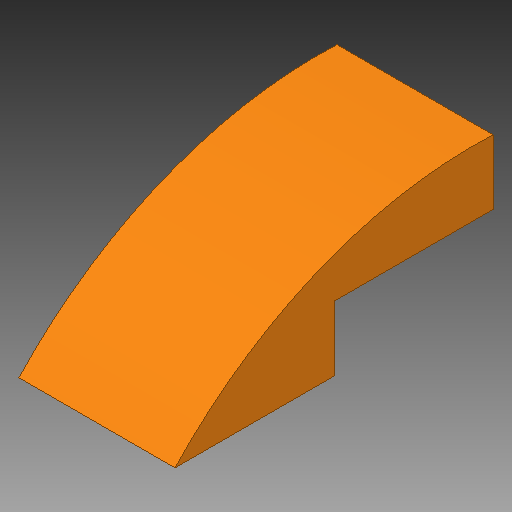
# Autodesk Inventor part: 2x1 curve
Saved by Autodesk Inventor 2017 (Build 210142000, 142)
## iProperties
Created: 2018-05-17
Part Number: 2x1 curve
Material: ABS Plastic
Document SubType Name: Modeling
Designer: 20000650
Density: 1.06 g/cm^3
Appearance: Orange
Mass: 0.311158 g
Surface Area: 4.69388 cm^2
Volume: 0.293546 cm^3
Author: 20000650
Autodesk Inventor part; units mm, degrees
ref_plane "YZ Plane" through (0, 0, 0) normal (1, 0, 0) x (0, 1, 0)
ref_plane "XZ Plane" through (0, 0, 0) normal (0, 1, 0) x (-1, 0, 0)
sketch "Sketch1" plane through (0, 0, 0) normal (1, 0, 0) x (0, 1, 0)
  line L0 (0, 0) -> (0, -7.9426)
  line L1 (0, -7.9426) -> (3.236, -7.9426)
  line L2 (3.236, -7.9426) -> (3.236, -15.8852)
  line L3 (3.236, -15.8852) -> (6.4618, -15.8852)
  arc A0 (6.4618, -15.8852) -> (0, 0) centre (-13.924, -14.9208) ccw
  dimension "d0" = 7.9426
  dimension "d1" = 3.236
  dimension "d2" = 7.9426
  dimension "d3" = 3.2258
  constraints: 8 end point, 3 perpendicular, 2 point on circle, 1 centre point, 1 vertical
  measures "d0" distance of L0.start L0.end
  measures "d1" distance of L0.end L1.end
  measures "d2" distance of L1.end L2.end
  measures "d3" distance of L2.end L3.end
extrude "Extrusion1" add sketch "Sketch1" along normal blind 7.7978
shell "Shell1" thickness 1.4732 removed faces 1 at (2.5993, 0, -2.6475)
ref_plane "Work Plane1" through (1.4732, 0, 0) normal (-1, 0, 0) x (0, 0, 1)
sketch "Sketch4" plane through (1.4732, 0, 0) normal (-1, 0, 0) x (0, 0, 1)
  line L0 (-7.9426, 3.236) -> (-15.8852, 3.236) projected
  line L1 (-15.8852, 3.236) -> (-15.8852, 6.4618) projected
  arc A0 (0, 0) -> (-15.8852, 6.4618) centre (-14.9208, -13.924) ccw projected
  line L2 (-14.412, 4.7092) -> (-14.412, 5.0045)
  arc A1 (-7.9426, 3.6786) -> (-14.412, 5.0045) centre (-14.9208, -13.924) ccw
  line L3 (-14.412, 5.0045) -> (-14.412, 3.236)
  line L4 (-7.9426, 3.236) -> (-15.8852, 3.236) projected
  line L5 (-7.9426, 3.236) -> (-7.9426, 3.6786)
  constraints: 6 end point, 2 point on circle, 1 centre point, 1 perpendicular, 1 point on line, 1 vertical
extrude "Extrusion2" cut sketch "Sketch4" against normal blind 4.8514
body "Solid1"
